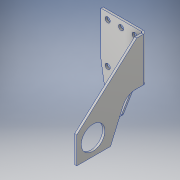
# Autodesk Inventor part: Roller bracket
Saved by Autodesk Inventor 2019 (Build 230136000, 136)
## iProperties
Created: 2018-11-09
Part Number: Roller bracket
Material: Aluminum 6061
Document SubType Name: Sheet Metal
Designer: woodk
Density: 2.7 g/cm^3
Sheet Metal Rule: Haakon
Appearance: Aluminum - Flat
Mass: 25.3313 g
Surface Area: 103.44 cm^2
Volume: 9.38197 cm^3
Author: woodk
Autodesk Inventor part; units mm, degrees
ref_plane "YZ Plane" through (0, 0, 0) normal (1, 0, 0) x (0, 1, 0)
ref_plane "XZ Plane" through (0, 0, 0) normal (0, 1, 0) x (-1, 0, 0)
ref_plane "XY Plane" through (0, 0, 0) normal (0, 0, 1) x (1, 0, 0)
sketch "Sketch1" plane through (0, 0, 0) normal (0, 0, 1) x (1, 0, 0)
  line L0 (0, 0) -> (41.275, 0)
  line L1 (41.275, 0) -> (41.275, 101.6)
  line L2 (41.275, 101.6) -> (0, 101.6)
  line L3 (0, 101.6) -> (0, 0)
  dimension "d0" = 101.6
  dimension "d1" = 41.275
  measures "d0" distance of L2.end L0.start
  measures "d1" distance of L0.start L0.end
extrude "Plate1" add sketch "Sketch1" along normal blind 2.032
sketch "Sketch2" plane through (39.243, 101.6, 0) normal (1, 0, 0) x (0, 1, 0)
  line L0 (-101.6, 0) -> (0, 0)
  line L1 (0, 0) -> (0, 66.04)
  line L2 (0, 66.04) -> (-101.6, 66.04)
  line L3 (-101.6, 66.04) -> (-101.6, 0)
  constraints: 6 end point, 1 horizontal, 1 perpendicular, 1 vertical
edge flange "Flange1" height 66.04 angle 90 thickness 2.032 bend radius 1.27 thickness toward (1, 0, 0) relief tear relief width 2.032 relief depth 1.016 edges at (41.275, 50.8, 2.032) wall of the first edge with corners at (39.243, 0, 0) (39.243, 101.6, 0) (39.243, 101.6, 66.04) (39.243, 0, 66.04)
bend "Bend1"
corner "Corner1"
sketch "Sketch3" plane through (0, 0, 2.032) normal (0, 0, 1) x (1, 0, 0)
  line L0 (0, 0) -> (0, 101.6) projected
  line L1 (0, 101.6) -> (37.973, 101.6) projected
  point P0 (6.35, 95.25)
  point P1 (6.35, 57.15)
  point P2 (19.05, 95.25)
  point P3 (31.75, 95.25)
  point P4 (19.05, 57.15)
  dimension "d13" = 6.35
  dimension "d14" = 6.35
  dimension "d15" = 38.1
  dimension "d16" = 12.7
  dimension "d17" = 12.7
  constraints: 3 horizontal alignment, 2 vertical alignment
  measures "d13" distance from line of L0 point (6.35, 95.25)
  measures "d14" distance from line of L1 point (6.35, 95.25)
  measures "d15" distance of point (6.35, 57.15) point (6.35, 95.25)
  measures "d16" distance of point (6.35, 95.25) point (19.05, 95.25)
  measures "d17" distance of point (19.05, 95.25) point (31.75, 95.25)
hole "Hole1" at (6.35, 95.25, 2.032) at (6.35, 57.15, 2.032) at (19.05, 95.25, 2.032) at (31.75, 95.25, 2.032) at (19.05, 57.15, 2.032) direction (0, 0, -1) diameter 4.8514 end through all
sketch "Sketch4" plane through (0, 0, 2.032) normal (0, 0, 1) x (1, 0, 0)
  line L0 (0, 101.6) -> (37.973, 101.6) projected
  line L1 (0, 0) -> (0, 101.6) projected
  point P0 (12.7, 26.6446)
  dimension "d25" = 74.9554
  dimension "d26" = 12.7
  measures "d25" distance from line of L0 point (12.7, 26.645)
  measures "d26" distance from line of L1 point (12.7, 26.645)
hole "Hole2" at (12.7, 26.6446, 2.032) direction (0, 0, -1) diameter 7.9375 end through all
sketch "Sketch5" plane through (0, 0, 2.032) normal (0, 0, 1) x (1, 0, 0)
  circle A0 centre (12.7, 26.6446) radius 3.9687 projected
  arc A1 (5.6431, 25.4938) -> (19.3942, 24.1322) centre (12.7, 26.6446) ccw
  line L0 (37.973, 101.6) -> (37.973, 0) projected
  line L1 (0, 101.6) -> (37.973, 101.6) projected
  line L2 (39.243, 101.6) -> (39.243, 0) projected
  line L3 (39.243, 60.0989) -> (32.893, 60.0989)
  line L4 (32.893, 60.0989) -> (19.3942, 24.1322)
  line L5 (0, 60.0989) -> (5.6431, 25.4938)
  line L6 (0, 0) -> (0, 101.6) projected
  line L7 (37.973, 0) -> (0, 0) projected
  line L8 (0, 60.0989) -> (0, 0)
  line L9 (0, 0) -> (39.243, 0)
  dimension "d34" = 14.3002
  dimension "d37" = 6.35
  dimension "d38" = 41.5011
  constraints: 10 end point, 2 point on circle, 2 point on line, 2 tangent, 1 centre point, 1 coincident, 1 horizontal, 1 horizontal alignment, 1 perpendicular, 1 vertical
  measures "d34" diameter of A1
  measures "d37" distance of L3.start L3.end
  measures "d38" distance between parallel lines of L1 L3
extrude "Extrusion1" cut sketch "Sketch5" against normal through all contours A1 L4 L3 L0 L7 L6 L5 | L3 L2 L9 L0
sketch "Sketch6" plane through (39.243, 0, 66.04) normal (-1, 0, 0) x (0, 0, 1)
  line L0 (-66.04, 101.6) -> (-66.04, 60.0989) projected
  line L1 (-62.738, 101.6) -> (0, 101.6) projected
  point P0 (-66.04, 0)
  point P1 (-15.24, 40.7924)
  dimension "d41" = 50.8
  dimension "d42" = 60.8076
  measures "d41" distance from line of L0 point (-15.24, 40.792)
  measures "d42" distance from line of L1 point (-15.24, 40.792)
hole "Hole3" at (39.243, 40.7924, 50.8) direction (1, 0, 0) diameter 22.225 end through all
sketch "Sketch7" plane through (39.243, 0, 66.04) normal (-1, 0, 0) x (0, 0, 1)
  line L0 (0, 0) -> (0, 101.6) projected
  line L1 (0, 25.4) -> (-31.75, 25.4)
  line L2 (-62.738, 101.6) -> (0, 101.6) projected
  line L3 (-64.008, 60.0989) -> (-65.786, 60.0989) projected
  line L4 (-65.786, 60.0989) -> (-46.736, 60.0989)
  line L5 (-31.75, 25.4) -> (-46.736, 60.0989)
  line L6 (0, 25.4) -> (0, 0)
  line L7 (-65.786, 0) -> (-65.786, 60.0989) projected
  line L8 (-65.786, 0) -> (-65.786, 60.0989)
  line L9 (0, 0) -> (-65.786, 0)
  point P0 (-66.04, 0)
  dimension "d50" = 76.2
  dimension "d51" = 31.75
  dimension "d54" = 19.05
  constraints: 12 end point, 3 horizontal, 2 collinear, 1 point on line
  measures "d50" distance between parallel lines of L1 L2
  measures "d51" distance of L1.start L1.end
  measures "d54" distance of L3.end L4.end
extrude "Extrusion2" cut sketch "Sketch7" against normal blind 6.35 and the other way blind 6.35
fillet "Fillet1" radius 12.7 1 edges at (40.259, 60.0989, 19.304)
sketch "Sketch8" plane through (39.243, 101.6, 3.302) normal (-1, 0, 0) x (0, 0, 1)
  line L0 (62.738, -76.2) -> (62.738, 0) projected
  line L1 (62.738, -50.8) -> (62.738, 0)
  line L2 (62.738, 0) -> (6.223, 0)
  line L3 (62.738, 0) -> (0, 0) projected
  line L4 (62.738, -50.8) -> (6.223, 0)
  line L5 (-3.302, 0) -> (-3.302, -41.5011) projected
  point P0 (-3.302, -101.6)
  dimension "d60" = 50.8
  dimension "d61" = 9.525
  constraints: 6 end point, 1 collinear, 1 point on line
  measures "d60" distance of L0.end L1.start
  measures "d61" distance from line of L5 L2.end
extrude "Extrusion3" cut sketch "Sketch8" against normal through all
equation "\"d23\" = Thickness"
equation "\"d32\" = Thickness"
equation "\"d48\" = Thickness"
equation "\"d2\" = Thickness"
equation "\"d3\" = BendReliefWidth"
equation "\"d4\" = BendReliefDepth"
equation "\"d5\" = MinimumRemnant"
equation "\"d6\" = TransitionRadius"
equation "\"d9\" = BendRadius"
equation "\"d10\" = CornerReliefSize"
equation "\"d11\" = GapSize"
equation "\"d12\" = JacobiRadiusSize"
equation "\"BendReliefWidth\" = Thickness"
equation "\"BendReliefDepth\" = 0.5 * Thickness"
equation "\"CornerReliefSize\" = 4 * Thickness"
equation "\"MinimumRemnant\" = 2 * Thickness"
equation "\"TransitionRadius\" = BendRadius"
equation "\"JacobiRadiusSize\" = BendRadius"
equation "\"GapSize\" = Thickness"
equation "\"Thickness\" = 2.032"
equation "\"BendRadius\" = 1.27"
body "Solid1"
